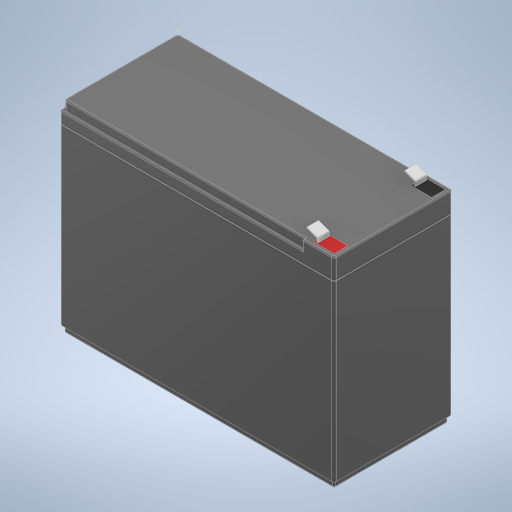
# Autodesk Inventor part: 12V Battery
Saved by Autodesk Inventor 2023 (Build 270158000, 158)
## iProperties
Created: 2022-07-12
Part Number: 12V Battery
Material: Generic
Document SubType Name: Modeling
Designer: justi
Density: 1 g/cm^3
Appearance: 0,0,0
Author: justi
Autodesk Inventor part; units mm, degrees
ref_plane "YZ Plane" through (0, 0, 0) normal (1, 0, 0) x (0, 1, 0)
ref_plane "XZ Plane" through (0, 0, 0) normal (0, 1, 0) x (-1, 0, 0)
ref_plane "XY Plane" through (0, 0, 0) normal (0, 0, 1) x (1, 0, 0)
sketch "Sketch1" plane through (0, 0, 0) normal (0, 0, 1) x (1, 0, 0)
  line L0 (0, 0) -> (150.876, 0)
  line L1 (150.876, 0) -> (150.876, 110.998)
  line L2 (150.876, 110.998) -> (0, 110.998)
  line L3 (0, 110.998) -> (0, 0)
  dimension "d0" = 110.998
  dimension "d1" = 150.876
  constraints: 8 end point, 2 parallel, 1 horizontal, 1 perpendicular
  measures "d0" distance of L2.end L0.start
  measures "d1" distance of L0.start L0.end
extrude "Extrusion1" add sketch "Sketch1" along normal blind 65.024
sketch "Sketch2" plane through (0, 0, 65.024) normal (0, 0, 1) x (1, 0, 0)
  point P0 (0, 0)
fillet "Fillet1" radius 1.27 4 edges at (150.876, 55.499, 65.024) (150.876, 55.499, 0) (0, 55.499, 65.024) (0, 55.499, 0)
sketch "Sketch3" plane through (0, 0, 65.024) normal (0, 0, 1) x (1, 0, 0)
  line L0 (1.27, 0) -> (0, 0) projected
  line L1 (150.876, 110.998) -> (150.876, 0) projected
  line L2 (0, 0) -> (150.876, 0)
  line L3 (150.876, 0) -> (150.876, 3.81)
  line L4 (150.876, 3.81) -> (0, 3.81)
  line L5 (0, 3.81) -> (0, 0)
  dimension "d5" = 3.81
  constraints: 8 end point, 2 parallel, 1 horizontal, 1 perpendicular, 1 point on line
  measures "d5" distance between parallel lines of L2 L4
extrude "Extrusion2" cut sketch "Sketch3" against normal blind 1.27
sketch "Sketch4" plane through (150.876, 0, 1.27) normal (1, 0, 0) x (0, 0, -1)
  line L0 (0, 0) -> (-62.484, 0) projected
  line L1 (-62.484, 0) -> (7.9509, 0)
  line L2 (7.9509, 0) -> (7.9509, 3.81)
  line L3 (7.9509, 3.81) -> (-62.484, 3.81)
  line L4 (-62.484, 3.81) -> (-62.484, 0)
  point P0 (1.27, 0)
  dimension "d8" = 3.81
  constraints: 8 end point, 2 parallel, 1 horizontal, 1 perpendicular
  measures "d8" distance of L1.end L2.end
extrude "Extrusion3" cut sketch "Sketch4" against normal blind 1.27
sketch "Sketch5" plane through (0, 0, 0) normal (0, 0, -1) x (-1, 0, 0)
  line L0 (-1.27, 0) -> (-149.606, 0) projected
  line L1 (-149.606, 0) -> (4.3491, 0)
  line L2 (4.3491, 0) -> (4.3491, 3.81)
  line L3 (4.3491, 3.81) -> (-149.606, 3.81)
  line L4 (-149.606, 3.81) -> (-149.606, 0)
  point P0 (0, 0)
  dimension "d11" = 3.81
  constraints: 8 end point, 2 parallel, 1 horizontal, 1 perpendicular
  measures "d11" distance of L1.end L2.end
extrude "Extrusion4" cut sketch "Sketch5" against normal blind 1.27
sketch "Sketch6" plane through (0, 110.998, 1.27) normal (-1, 0, 0) x (0, 0, 1)
  line L0 (-2.7889, -110.998) -> (77.0099, -110.998)
  line L1 (77.0099, -110.998) -> (77.0099, -107.188)
  line L2 (77.0099, -107.188) -> (-2.7889, -107.188)
  line L3 (-2.7889, -107.188) -> (-2.7889, -110.998)
  point P0 (-1.27, -110.998)
  dimension "d14" = 3.81
  constraints: 8 end point, 2 parallel, 1 horizontal, 1 perpendicular
  measures "d14" distance of L0.end L1.end
extrude "Extrusion5" cut sketch "Sketch6" against normal blind 1.27
fillet "Fillet2" radius 0.635 8 edges at (1.27, 1.905, 1.27) (75.438, 0, 1.27) (1.27, 0, 32.512) (1.27, 1.905, 63.754) (75.438, 0, 63.754) (149.606, 1.905, 63.754) (149.606, 0, 32.512) (149.606, 1.905, 1.27)
sketch "Sketch7" plane through (0, 0, 65.024) normal (0, 0, 1) x (1, 0, 0)
  line L0 (0, 110.998) -> (1.27, 110.998) projected
  line L1 (0, 110.998) -> (133.35, 110.998)
  line L2 (133.35, 110.998) -> (133.35, 105.918)
  line L3 (133.35, 105.918) -> (0, 105.918)
  line L4 (0, 105.918) -> (0, 110.998)
  point P0 (0, 0)
  dimension "d18" = 133.35
  dimension "d19" = 5.08
  constraints: 8 end point, 2 parallel, 1 horizontal, 1 perpendicular
  measures "d18" distance of L2.end L3.end
  measures "d19" distance of L1.end L2.end
extrude "Extrusion6" cut sketch "Sketch7" against normal blind 1.27
sketch "Sketch8" plane through (0, 3.81, 1.27) normal (-1, 0, 0) x (0, 0, 1)
  line L0 (62.484, 107.188) -> (62.484, 102.108) projected
  line L1 (62.484, 107.188) -> (-1.9626, 107.188)
  line L2 (-1.9626, 107.188) -> (-1.9626, 102.108)
  line L3 (-1.9626, 102.108) -> (62.484, 102.108)
  line L4 (62.484, 102.108) -> (62.484, 107.188)
  point P0 (-1.27, -3.81)
  constraints: 8 end point, 2 parallel, 1 horizontal, 1 perpendicular
extrude "Extrusion7" cut sketch "Sketch8" against normal blind 1.27
sketch "Sketch9" plane through (0, 0, 0) normal (0, 0, -1) x (-1, 0, 0)
  line L0 (-149.606, 110.998) -> (-1.27, 110.998) projected
  line L1 (-1.27, 110.998) -> (-134.62, 110.998)
  line L2 (-134.62, 110.998) -> (-134.62, 105.918)
  line L3 (-134.62, 105.918) -> (-1.27, 105.918)
  line L4 (-1.27, 105.918) -> (-1.27, 110.998)
  point P0 (0, 0)
  dimension "d24" = 133.35
  dimension "d25" = 5.08
  constraints: 8 end point, 2 parallel, 1 horizontal, 1 perpendicular
  measures "d24" distance of L2.end L3.end
  measures "d25" distance of L1.end L2.end
extrude "Extrusion8" cut sketch "Sketch9" against normal blind 1.27
sketch "Sketch10" plane through (0, 0, 0) normal (0, 0, -1) x (-1, 0, 0)
  line L0 (-150.876, 3.81) -> (-150.876, 110.998) projected
  line L1 (-150.876, 99.568) -> (14.4138, 99.568)
  line L2 (14.4138, 99.568) -> (14.4138, 99.314)
  line L3 (14.4138, 99.314) -> (-150.876, 99.314)
  line L4 (-150.876, 99.314) -> (-150.876, 99.568)
  line L5 (-149.606, 110.998) -> (-134.62, 110.998) projected
  point P0 (0, 0)
  dimension "d28" = 11.43
  dimension "d29" = 0.254
  constraints: 8 end point, 2 parallel, 1 horizontal, 1 perpendicular, 1 point on line
  measures "d28" distance between parallel lines of L5 L1
  measures "d29" distance of L1.end L2.end
extrude "Extrusion9" cut sketch "Sketch10" against normal blind 0.635
sketch "Sketch11" plane through (0, 3.81, 1.27) normal (-1, 0, 0) x (0, 0, 1)
  line L0 (-0.635, 95.758) -> (68.672, 95.758)
  line L1 (68.672, 95.758) -> (68.672, 95.504)
  line L2 (68.672, 95.504) -> (-0.635, 95.504)
  line L3 (-0.635, 95.504) -> (-0.635, 95.758)
  point P0 (-1.27, -3.81)
  dimension "d32" = 0.254
  constraints: 8 end point, 2 parallel, 1 horizontal, 1 perpendicular
  measures "d32" distance of L0.end L1.end
extrude "Extrusion10" cut sketch "Sketch11" against normal blind 0.635
sketch "Sketch12" plane through (0, 0, 65.024) normal (0, 0, 1) x (1, 0, 0)
  line L0 (0.635, 99.568) -> (0.635, 99.314) projected
  line L1 (0.635, 99.568) -> (153.0152, 99.568)
  line L2 (153.0152, 99.568) -> (153.0152, 99.314)
  line L3 (153.0152, 99.314) -> (0.635, 99.314)
  line L4 (0.635, 99.314) -> (0.635, 99.568)
  point P0 (0, 0)
  constraints: 8 end point, 2 parallel, 1 horizontal, 1 perpendicular
extrude "Extrusion11" cut sketch "Sketch12" against normal blind 0.635
sketch "Sketch13" plane through (150.876, 110.998, 63.754) normal (1, 0, 0) x (0, 0, -1)
  line L0 (-0.635, -11.684) -> (-0.635, -11.43) projected
  line L1 (-0.635, -11.43) -> (64.1446, -11.43)
  line L2 (64.1446, -11.43) -> (64.1446, -11.684)
  line L3 (64.1446, -11.684) -> (-0.635, -11.684)
  line L4 (-0.635, -11.684) -> (-0.635, -11.43)
  point P0 (63.754, -110.998)
  constraints: 8 end point, 2 parallel, 1 horizontal, 1 perpendicular
extrude "Extrusion12" cut sketch "Sketch13" against normal blind 0.635
fillet "Fillet3" radius 0.635 17 edges at (0.372, 105.918, 64.652) (0, 105.918, 32.512) (0.372, 105.918, 0.372) (67.945, 105.918, 0) (67.31, 105.918, 65.024) (133.35, 108.458, 65.024) (67.31, 110.998, 63.754) (1.27, 110.998, 32.512) (67.945, 110.998, 1.27) (134.62, 108.458, 0) (134.62, 110.998, 0.635) (150.504, 110.998, 0.372) (150.876, 110.998, 32.512) (150.504, 110.998, 64.652) (141.478, 110.998, 65.024) (142.113, 110.998, 0) (133.35, 110.998, 64.389)
fillet "Fillet4" radius 1.27 4 edges at (1.456, 110.812, 1.456) (1.27, 108.1405, 1.27) (1.456, 110.812, 63.568) (1.27, 108.1405, 63.754)
sketch "Sketch14" plane through (133.985, 110.998, 64.389) normal (0, 1, 0) x (1, 0, 0)
  line L0 (15.621, 1.27) -> (14.986, 1.27) projected
  line L1 (14.986, 1.27) -> (3.556, 1.27)
  line L2 (3.556, 1.27) -> (3.556, 8.89)
  line L3 (3.556, 8.89) -> (14.986, 8.89)
  line L4 (14.986, 8.89) -> (14.986, 1.27)
  line L5 (14.986, 1.27) -> (14.986, 62.484) projected
  line L6 (14.986, 62.484) -> (3.556, 62.484)
  line L7 (3.556, 62.484) -> (3.556, 54.864)
  line L8 (3.556, 54.864) -> (14.986, 54.864)
  line L9 (14.986, 54.864) -> (14.986, 62.484)
  point P0 (-133.985, 64.389)
  point P1 (14.986, 54.864)
  dimension "d41" = 11.43
  dimension "d42" = 7.62
  dimension "d43" = 7.62
  constraints: 16 end point, 4 parallel, 2 horizontal, 2 perpendicular
  measures "d41" distance of L2.end L3.end
  measures "d42" distance of L1.end L2.end
  measures "d43" distance of L6.end L7.end
sketch "Sketch15" plane through (133.985, 110.998, 64.389) normal (0, 1, 0) x (1, 0, 0)
  point P0 (-133.985, 64.389)
extrude "Extrusion13" cut sketch "Sketch14" against normal blind 0.0254
sketch "Sketch16" plane through (133.985, 110.9726, 64.389) normal (0, 1, 0) x (1, 0, 0)
  line L0 (5.461, 1.905) -> (4.826, 1.905)
  line L1 (4.826, 1.905) -> (4.826, 8.255)
  line L2 (4.826, 8.255) -> (5.461, 8.255)
  line L3 (5.461, 8.255) -> (5.461, 1.905)
  line L4 (14.986, 1.27) -> (3.556, 1.27) projected
  line L5 (3.556, 1.27) -> (3.556, 8.89) projected
  point P0 (-133.985, 64.389)
  dimension "d46" = 0.635
  dimension "d47" = 6.35
  dimension "d48" = 0.635
  dimension "d49" = 1.27
  constraints: 8 end point, 2 parallel, 1 horizontal, 1 perpendicular
  measures "d46" distance of L1.end L2.end
  measures "d47" distance of L0.end L1.end
  measures "d48" distance between parallel lines of L4 L0
  measures "d49" distance between parallel lines of L5 L1
extrude "Extrusion14" add sketch "Sketch16" along normal blind 2.54
sketch "Sketch17" plane through (133.985, 110.998, 64.389) normal (0, 1, 0) x (1, 0, 0)
  point P0 (-133.985, 64.389)
sketch "Sketch18" plane through (133.985, 110.9726, 64.389) normal (0, 1, 0) x (1, 0, 0)
  line L0 (5.461, 55.499) -> (4.826, 55.499)
  line L1 (4.826, 55.499) -> (4.826, 61.849)
  line L2 (4.826, 61.849) -> (5.461, 61.849)
  line L3 (5.461, 61.849) -> (5.461, 55.499)
  line L4 (3.556, 54.864) -> (3.556, 62.484) projected
  line L5 (14.986, 54.864) -> (3.556, 54.864) projected
  point P0 (-133.985, 64.389)
  dimension "d52" = 0.635
  dimension "d53" = 1.27
  dimension "d54" = 0.635
  dimension "d55" = 6.35
  constraints: 8 end point, 2 parallel, 1 horizontal, 1 perpendicular
  measures "d52" distance of L1.end L2.end
  measures "d53" distance between parallel lines of L4 L1
  measures "d54" distance between parallel lines of L5 L0
  measures "d55" distance of L0.end L1.end
extrude "Extrusion15" add sketch "Sketch18" along normal blind 2.54
sketch "Sketch19" plane through (139.446, 110.9726, 56.134) normal (0, 0, -1) x (-1, 0, 0)
  line L0 (0, 2.54) -> (0.635, 2.54) projected
  line L1 (0, 2.54) -> (5.967, 4.7118)
  line L2 (5.967, 4.7118) -> (0, 2.54)
  line L3 (0, 2.54) -> (0.2172, 1.9433)
  line L4 (0.2172, 1.9433) -> (6.1842, 4.1151)
  line L5 (6.1842, 4.1151) -> (5.967, 4.7118)
  point P0 (139.446, -110.9726)
  dimension "d58" = 6.35
  dimension "d59" = 20
  dimension "d60" = 0.635
  constraints: 10 end point, 3 equal length, 1 perpendicular
  measures "d58" distance of L0.start L1.end
  measures "d59" angle of L1 L0
  measures "d60" distance of L3.end L0.start
extrude "Extrusion16" add sketch "Sketch19" against normal blind 6.35
sketch "Sketch20" plane through (139.446, 110.9726, 2.54) normal (0, 0, -1) x (-1, 0, 0)
  line L0 (0, 2.54) -> (0.635, 2.54) projected
  line L1 (0, 2.54) -> (5.967, 4.7118) projected
  line L2 (0, 2.54) -> (5.967, 4.7118)
  line L3 (5.967, 4.7118) -> (6.1842, 4.1151) projected
  line L4 (0, 2.54) -> (5.967, 4.7118)
  line L5 (5.967, 4.7118) -> (6.1842, 4.1151)
  line L6 (6.1842, 4.1151) -> (0.2172, 1.9433)
  line L7 (0.2172, 1.9433) -> (0, 2.54)
  point P0 (139.446, -110.9726)
  constraints: 10 end point, 3 equal length, 2 perpendicular
extrude "Extrusion17" add sketch "Sketch20" against normal blind 6.35
body "Solid1"
